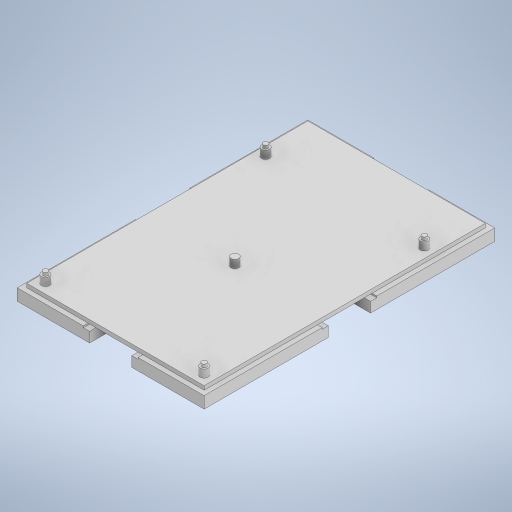
# Autodesk Inventor part: Base
Saved by Autodesk Inventor 2023 (Build 270158000, 158)
## iProperties
Created: 2023-01-13
Part Number: Base
Material: Generic
Document SubType Name: Modeling
Designer: Ahmed Nazir
Density: 1 g/cm^3
Appearance: Default
Author: Ahmed Nazir
Autodesk Inventor part; units mm, degrees
ref_plane "YZ Plane" through (0, 0, 0) normal (1, 0, 0) x (0, 1, 0)
ref_plane "XZ Plane" through (0, 0, 0) normal (0, 1, 0) x (-1, 0, 0)
ref_plane "XY Plane" through (0, 0, 0) normal (0, 0, 1) x (1, 0, 0)
sketch "Sketch1" plane through (0, 0, 0) normal (0, 1, 0) x (-1, 0, 0)
  line L0 (0, 0) -> (113.6, 0)
  line L1 (113.6, 0) -> (113.6, -180)
  line L2 (113.6, -180) -> (0, -180)
  line L3 (0, -180) -> (0, 0)
  line L4 (116.6, -183) -> (116.6, 3)
  line L5 (116.6, 3) -> (-3, 3)
  line L6 (-3, 3) -> (-3, -183)
  line L7 (-3, -183) -> (116.6, -183)
  circle A0 centre (6, -6) radius 1.6
  circle A1 centre (6, -6) radius 2.6
  circle A2 centre (56.8, -76.485) radius 2.5
  circle A3 centre (6, -146.97) radius 1.6
  circle A4 centre (6, -146.97) radius 2.6
  circle A5 centre (107.6, -6) radius 1.6
  circle A6 centre (107.6, -6) radius 2.6
  circle A7 centre (107.6, -146.97) radius 1.6
  circle A8 centre (107.6, -146.97) radius 2.6
  dimension "d0" = 113.6
  dimension "d1" = 180
  dimension "d2" = 3
  dimension "d22" = 3.2
  dimension "d23" = 1
  dimension "d24" = 6
  dimension "d25" = 6
  dimension "d26" = 5
  dimension "d35" = 3.2
  dimension "d36" = 1
  dimension "d37" = 140.97
  dimension "d38" = 0
  dimension "d39" = 3.2
  dimension "d40" = 1
  dimension "d41" = 101.6
  dimension "d42" = 0
  dimension "d43" = 3.2
  dimension "d44" = 1
  dimension "d45" = 0
  dimension "d46" = 0
  dimension "d47" = 50.8
  dimension "d48" = 70.485
  constraints: 16 end point, 9 centre point, 4 parallel, 2 perpendicular, 1 horizontal, 3 other
  measures "d0" distance of L1.end L2.end
  measures "d1" distance of L0.end L1.end
  measures "d2" distance between parallel lines of L1 L4
  measures "d22" diameter of A0
  measures "d23" radial gap between concentric circles of A0 A1
  measures "d24" distance from line of L3 A0.centre
  measures "d25" distance from line of A0.centre L0
  measures "d26" diameter of A2
  measures "d35" diameter of A3
  measures "d36" radial gap between concentric circles of A3 A4
  measures "d37" distance of A3.centre A0.centre
  measures "d38" horizontal distance of A3.centre A0.centre
  measures "d39" diameter of A5
  measures "d40" radial gap between concentric circles of A5 A6
  measures "d41" distance of A0.centre A5.centre
  measures "d42" vertical distance of A5.centre A0.centre
  measures "d43" diameter of A7
  measures "d44" radial gap between concentric circles of A7 A8
  measures "d45" vertical distance of A3.centre A7.centre
  measures "d46" horizontal distance of A5.centre A7.centre
  measures "d47" horizontal distance of A2.centre A0.centre
  measures "d48" vertical distance of A2.centre A5.centre
extrude "Extrusion13" add sketch "Sketch1" along normal blind 10 contours L0 L1 L2 L3 | A0 | A1 | A2 | A3 | A4 | A5 | A6 | A7 | A8
extrude "Extrusion14" add sketch "Sketch1" along normal blind 7.5 contours L7 L6 L5 L4
sketch "Sketch6" plane through (0, 10, 0) normal (0, 1, 0) x (1, 0, 0)
  circle A0 centre (-107.6, 6) radius 2.6 projected
  circle A1 centre (-107.6, 6) radius 1.6 projected
  circle A2 centre (-6, 6) radius 2.6 projected
  circle A3 centre (-6, 6) radius 1.6 projected
  circle A4 centre (-6, 146.97) radius 2.6 projected
  circle A5 centre (-6, 146.97) radius 1.6 projected
  circle A6 centre (-107.6, 146.97) radius 2.6 projected
  circle A7 centre (-107.6, 146.97) radius 1.6 projected
  circle A8 centre (-56.8, 76.485) radius 2.5 projected
  point P0 (0, 0)
extrude "Extrusion15" add sketch "Sketch6" along normal blind 7 contours A1 | A3 | A5 | A7
extrude "Extrusion16" add sketch "Sketch6" along normal blind 5
sketch "Sketch8" plane through (-116.6, 0, 3) normal (0, 0, 1) x (1, 0, 0)
  line L0 (119.6, 0) -> (0, 0) projected
  line L1 (59.8, 0) -> (59.8, 10)
  line L2 (3, 10) -> (116.6, 10) projected
  line L3 (59.8, 7.5) -> (42.3, 7.5)
  line L4 (42.3, 7.5) -> (42.3, 6.5)
  line L5 (42.3, 6.5) -> (46.3, 6.5)
  line L6 (46.3, 6.5) -> (46.3, 0)
  line L7 (46.3, 0) -> (59.8, 0)
  line L8 (59.8, 7.5) -> (77.3, 7.5)
  line L9 (77.3, 7.5) -> (77.3, 6.5)
  line L10 (77.3, 6.5) -> (73.3, 6.5)
  line L11 (73.3, 6.5) -> (73.3, 0)
  line L12 (73.3, 0) -> (59.8, 0)
  point P0 (116.6, 0)
  point P1 (73.3, 0)
  dimension "d116" = 17.5
  dimension "d117" = 1
  dimension "d118" = 4
  dimension "d119" = 7.5
  constraints: 22 end point, 4 perpendicular, 4 symmetric about line, 2 midpoint, 2 point on line, 1 parallel
  measures "d116" distance of L3.start L3.end
  measures "d117" distance of L3.end L4.end
  measures "d118" distance of L4.end L5.end
  measures "d119" distance between parallel lines of L0 L3
sketch "Sketch7" plane through (3, 0, 3) normal (1, 0, 0) x (0, 0, -1)
  line L0 (0, 0) -> (186, 0) projected
  line L1 (93, 0) -> (93, 10)
  line L2 (183, 10) -> (3, 10) projected
  line L3 (79.5, 6.5) -> (75.5, 6.5)
  line L4 (79.5, 6.5) -> (79.5, 0)
  line L5 (79.5, 0) -> (93, 0)
  line L6 (75.5, 6.5) -> (75.5, 7.5)
  line L7 (75.5, 7.5) -> (93, 7.5)
  line L8 (106.5, 6.5) -> (110.5, 6.5)
  line L9 (106.5, 6.5) -> (106.5, 0)
  line L10 (106.5, 0) -> (93, 0)
  line L11 (110.5, 6.5) -> (110.5, 7.5)
  line L12 (110.5, 7.5) -> (93, 7.5)
  point P0 (3, 0)
  point P1 (86.25, 0)
  point P2 (99.75, 0)
  point P3 (79.5, 0)
  point P4 (106.5, 0)
  dimension "d108" = 4
  dimension "d110" = 27
  dimension "d112" = 1
  dimension "d113" = 7.5
  constraints: 22 end point, 5 symmetric about line, 3 midpoint, 3 point on line, 2 perpendicular, 2 vertical, 1 horizontal
  measures "d108" distance of L3.start L3.end
  measures "d110" diameter of L4 L1
  measures "d112" distance of L3.end L6.end
  measures "d113" distance between parallel lines of L0 L7
extrude "Extrusion18" cut sketch "Sketch8" against normal through all
extrude "Extrusion19" cut sketch "Sketch7" against normal through all
body "Solid2"
